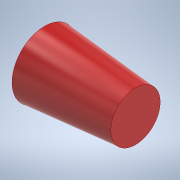
# Autodesk Inventor part: Conical rubber plug 12mm
Saved by Autodesk Inventor 2020 (Build 240168000, 168)
## iProperties
Created: 2020-07-11
Part Number: Conical rubber plug 12mm
Material: Rubber
Document SubType Name: Modeling
Designer: Bruno
Density: 0.93 g/cm^3
Appearance: Red
Author: Bruno
Autodesk Inventor part; units mm, degrees
ref_plane "YZ Plane" through (0, 0, 0) normal (1, 0, 0) x (0, 1, 0)
ref_plane "XZ Plane" through (0, 0, 0) normal (0, 1, 0) x (-1, 0, 0)
ref_plane "XY Plane" through (0, 0, 0) normal (0, 0, 1) x (1, 0, 0)
sketch "Sketch1" plane through (0, 0, 0) normal (0, 1, 0) x (-1, 0, 0)
  line L0 (0, 0) -> (0, 4.75)
  line L1 (0, 0) -> (17.5, 0)
  line L2 (17.5, 0) -> (17.5, 6.25)
  line L3 (17.5, 6.25) -> (0, 4.75)
  dimension "d0" = 4.75
  dimension "d1" = 17.5
  dimension "d2" = 6.25
  constraints: 8 end point, 1 horizontal, 1 perpendicular, 1 vertical
  measures "d0" distance of L0.start L0.end
  measures "d1" distance of L0.start L1.end
  measures "d2" distance of L1.end L2.end
revolve "Revolution1" add sketch "Sketch1" angle 360 about axis through (0, 0, 0) along (-1, 0, 0)
body "Solid1"
